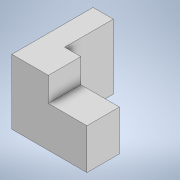
# Autodesk Inventor part: lab1ex1
Saved by Autodesk Inventor 2021 (Build 250183000, 183)
## iProperties
Created: 2022-02-28
Part Number: lab1ex1
Material: Generic
Document SubType Name: Modeling
Designer: Admin
Density: 1 g/cm^3
Appearance: Default
Author: Admin
Autodesk Inventor part; units mm, degrees
ref_plane "YZ Plane" through (0, 0, 0) normal (1, 0, 0) x (0, 1, 0)
ref_plane "XZ Plane" through (0, 0, 0) normal (0, 1, 0) x (-1, 0, 0)
ref_plane "XY Plane" through (0, 0, 0) normal (0, 0, 1) x (1, 0, 0)
sketch "Sketch1" plane through (0, 0, 0) normal (1, 0, 0) x (0, 1, 0)
  point P0 (0, 0)
sketch "Sketch2" plane through (0, 0, 0) normal (1, 0, 0) x (0, 1, 0)
  line L0 (32, 8.5828) -> (0, 8.5828)
  line L1 (0, 8.5828) -> (0, -31.4172)
  line L2 (0, -31.4172) -> (32, -31.4172)
  line L3 (32, -31.4172) -> (32, 8.5828)
  point P0 (0, 0)
  dimension "d0" = 32
  dimension "d1" = 40
  constraints: 8 end point, 2 parallel, 1 horizontal, 1 perpendicular
  measures "d0" distance of L1.end L2.end
  measures "d1" distance of L0.end L1.end
extrude "Extrusion1" add sketch "Sketch2" along normal blind 10
sketch "Sketch3" plane through (10, 0, 0) normal (1, 0, 0) x (0, 0, -1)
  point P0 (0, 0)
sketch "Sketch4" plane through (10, 0, 0) normal (1, 0, 0) x (0, 0, -1)
  line L0 (-8.5828, 32) -> (-8.5828, 0) projected
  line L1 (-8.5828, 0) -> (31.4172, 0) projected
  line L2 (-8.5828, 32) -> (7.4172, 32)
  line L3 (7.4172, 32) -> (7.4172, 0)
  line L4 (7.4172, 0) -> (-8.5828, 0)
  line L5 (-8.5828, 0) -> (-8.5828, 32)
  point P0 (0, 0)
  dimension "d4" = 16
  constraints: 8 end point, 2 parallel, 1 horizontal, 1 perpendicular, 1 point on line
  measures "d4" distance of L0.start L2.end
extrude "Extrusion2" add sketch "Sketch4" along normal blind 8
sketch "Sketch5" plane through (18, 0, 0) normal (1, 0, 0) x (0, 0, -1)
  line L0 (-8.5828, 32) -> (-8.5828, 0) projected
  line L1 (-8.5828, 0) -> (31.4172, 0) projected
  line L2 (-8.5828, 20) -> (7.4172, 20)
  line L3 (7.4172, 20) -> (7.4172, 0)
  line L4 (7.4172, 0) -> (-8.5828, 0)
  line L5 (-8.5828, 0) -> (-8.5828, 20)
  point P0 (0, 0)
  dimension "d7" = 16
  dimension "d8" = 20
  constraints: 8 end point, 2 parallel, 2 point on line, 1 horizontal, 1 perpendicular
  measures "d7" distance of L2.start L2.end
  measures "d8" distance of L2.end L3.end
extrude "Extrusion3" add sketch "Sketch5" along normal blind 19
body "Solid1"
